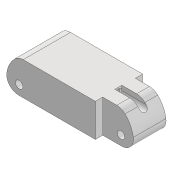
# Autodesk Inventor part: Distal_phalange
Saved by Autodesk Inventor 2022 (Build 260153000, 153)
## iProperties
Created: 2022-08-27
Part Number: Distal_phalange
Material: Generic
Document SubType Name: Modeling
Designer: dell
Density: 1 g/cm^3
Appearance: Default
Author: dell
Autodesk Inventor part; units mm, degrees
ref_plane "YZ Plane" through (0, 0, 0) normal (1, 0, 0) x (0, 1, 0)
ref_plane "XZ Plane" through (0, 0, 0) normal (0, 1, 0) x (-1, 0, 0)
ref_plane "XY Plane" through (0, 0, 0) normal (0, 0, 1) x (1, 0, 0)
sketch "Sketch1" plane through (0, 0, 0) normal (0, 0, 1) x (1, 0, 0)
  line L0 (0, 0) -> (-40, 0) construction
  line L1 (0, 10) -> (-40, 10)
  line L2 (-40, -10) -> (0, -10)
  arc A0 (0, -10) -> (0, 10) centre (0, 0) ccw
  arc A1 (-40, 10) -> (-40, -10) centre (-40, 0) ccw
  circle A2 centre (-40, 0) radius 1.55
  circle A3 centre (0, 0) radius 1.55
  line L3 (-40, 10) -> (0, 10)
  line L4 (0, 10) -> (0, 15)
  line L5 (0, 15) -> (-40, 15)
  line L6 (-40, 15) -> (-40, 10)
  line L7 (-49.1652, -4) -> (9.1652, -4)
  arc A4 (-40, 10) -> (-40, -10) centre (-33.3668, 0) ccw
  arc A5 (0, -10) -> (0, 10) centre (-6.6332, 0) ccw
  point P0 (-20, 0)
  point P1 (-44.6805, -4)
  point P2 (4.6805, -4)
  dimension "d0" = 20
  dimension "d1" = 40
  dimension "d2" = 3.1
  dimension "d3" = 3.1
  dimension "d7" = 5
  dimension "d13" = 4
  dimension "d20" = 12
  dimension "d26" = 12
  constraints: 18 end point, 10 point on circle, 6 centre point, 4 equal length, 4 tangent, 2 coincident, 2 horizontal, 1 midpoint, 1 perpendicular
  measures "d0" diameter of A1
  measures "d1" distance of L0.end L0.start
  measures "d2" diameter of A2
  measures "d3" diameter of A3
  measures "d7" distance of L4.end L1.start
  measures "d13" distance from line of L0.end L7
  measures "d20" radius of A4
  measures "d26" radius of A5
extrude "Extrusion1" add sketch "Sketch1" along normal blind 20 contours A5 L7 A4 L1
sketch "Sketch3" plane through (0, 0, 0) normal (1, 0, 0) x (0, 1, 0)
  circle A0 centre (8, 10) radius 1
  line L0 (8, 10) -> (13.1893, 10) construction
  line L1 (8, 8.5) -> (13.1893, 8.5)
  line L2 (13.1893, 11.5) -> (8, 11.5)
  arc A1 (8, 11.5) -> (8, 8.5) centre (8, 10) ccw
  arc A2 (13.1893, 8.5) -> (13.1893, 11.5) centre (13.1893, 10) ccw
  point P0 (0, 0)
  point P1 (10.5947, 10)
  dimension "d8" = 2
  dimension "d9" = 8
  dimension "d10" = 10
  dimension "d31" = 3
  constraints: 8 end point, 4 point on circle, 4 tangent, 3 centre point, 1 horizontal, 1 midpoint, 1 parallel
  measures "d8" diameter of A0
  measures "d9" horizontal distance of point (0, 0) L0.start
  measures "d10" vertical distance of point (0, 0) L0.start
  measures "d31" diameter of A2
extrude "Extrusion2" cut sketch "Sketch3" along normal mid plane 200 contours A0
extrude "Extrusion5" cut sketch "Sketch3" along normal blind 10 and the other way blind 8
fillet "Fillet1" radius 5 5 edges at (-44.6805, -4, 10) (-40, 10, 10) (0, 10, 15.75) (0, 10, 4.25) (4.6805, -4, 10)
sketch "Sketch5" plane through (0, 10, 20) normal (0, 1, 0) x (1, 0, 0)
  line L0 (-40.295, 20) -> (4.6805, 20) projected
  line L1 (-30.295, 17) -> (-30.295, 3)
  line L2 (-30.295, 3) -> (-56.111, 3)
  line L3 (-56.111, 3) -> (-56.111, 17)
  line L4 (-56.111, 17) -> (-30.295, 17)
  line L5 (-38.45, 0) -> (-41.55, 0) projected
  line L6 (-38.45, 20) -> (-41.55, 20) projected
  line L7 (-40.295, 20) -> (-40.295, 0) projected
  line L8 (0, 0) -> (-38.2657, 0) projected
  line L9 (1.55, 0) -> (-1.55, 0) projected
  line L10 (1.55, 20) -> (-1.55, 20) projected
  line L11 (-7.705, 16.9) -> (8.295, 16.9)
  line L12 (8.295, 16.9) -> (8.295, 3.1)
  line L13 (8.295, 3.1) -> (-7.705, 3.1)
  line L14 (-7.705, 3.1) -> (-7.705, 16.9)
  line L15 (-40.295, 0) -> (0.295, 0) projected
  line L16 (0.295, 0) -> (0.295, 20) projected
  line L17 (-7.705, 16.9) -> (-7.705, 20)
  line L18 (-7.705, 20) -> (8.295, 20)
  line L19 (8.295, 20) -> (8.295, 16.9)
  line L20 (8.295, 16.9) -> (-7.705, 16.9)
  line L21 (-7.705, 3.1) -> (-7.705, 0)
  line L22 (-7.705, 0) -> (8.295, 0)
  line L23 (8.295, 0) -> (8.295, 3.1)
  line L24 (8.295, 3.1) -> (-7.705, 3.1)
  point P0 (0, 20)
  point P1 (8.295, 3.1)
  point P2 (0, 0)
  point P3 (8.295, 16.9)
  point P4 (4.6805, 20)
  dimension "d21" = 10
  dimension "d22" = 3
  dimension "d23" = 3
  dimension "d27" = 3.1
  dimension "d28" = 3.1
  dimension "d29" = 8
  constraints: 32 end point, 8 parallel, 4 perpendicular, 3 point on line, 2 vertical
  measures "d21" distance between parallel lines of L7 L1
  measures "d22" distance between parallel lines of L0 L4
  measures "d23" distance between parallel lines of L8 L2
  measures "d27" distance between parallel lines of L8 L13
  measures "d28" distance between parallel lines of L0 L11
  measures "d29" distance between parallel lines of L16 L14
extrude "Extrusion4" cut sketch "Sketch5" against normal blind 200 contours L0 L16 L11 L17 | L0 L18 L19 L11 L16 | L13 L16 L9 L8 L21 | L13 L23 L22 L9 L16
fillet "Fillet2" radius 0.5 1 edges at (-8, 7, 10)
body "Solid1"
